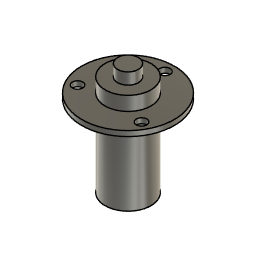
Slew_Bearing (Autodesk Fusion 360 archive; units mm, degrees)
design "GOCO bearing"
Autodesk Fusion 360 part; units mm, degrees
sketch "Sketch1" plane through (0, 0, 0) normal (0, 0, 1) x (1, 0, 0)
  circle A0 centre (0, 0) radius 22.25
  line L0 (0, 0) -> (0, 22.25) construction
  circle A1 centre (0, 17.75) radius 2.5
  line L1 (0, 17.75) -> (0, 20.25) construction
  circle A2 centre (-15.372, -8.875) radius 2.5
  circle A3 centre (15.372, -8.875) radius 2.5
  circle A4 centre (0, 0) radius 17.75 construction
  dimension "d1" = 44.5
  dimension "d2" = 5
  dimension "d3" = 2
  dimension "d5" = 360
  constraint coincident A0.centre L0.start
  constraint coincident A0 L0.end
  constraint vertical L0
  constraint coincident L0 A1.centre
  constraint coincident A1.centre L1.start
  constraint coincident L0 L1.end
  constraint coincident A1 L1.end
  constraint coincident A1.centre A4
  measures "d1" diameter of A0
  measures "d2" diameter of A1
  measures "d3" distance of L0.end L1.end
extrude "Extrude1" add sketch "Sketch1" along normal blind 2.5 makes body 1
sketch "Sketch2" plane through (0, 0, 2.5) normal (0, 0, 1) x (-1, 0, 0)
  circle A0 centre (0, -17.75) radius 2.5
  circle A1 centre (15.372, 8.875) radius 2.5
  circle A2 centre (-15.372, 8.875) radius 2.5
  circle A3 centre (0, 0) radius 22.25
  circle A4 centre (0, 0) radius 11
  dimension "d8" = 22
  constraint coincident A3.centre A4.centre
  measures "d8" diameter of A4
extrude "Extrude2" add sketch "Sketch2" along normal blind 6.7 contours A4 bodies 1
sketch "Sketch3" plane through (0, 0, 9.2) normal (0, 0, 1) x (-1, 0, 0)
  circle A0 centre (0, 0) radius 11
  circle A1 centre (0, 0) radius 5
  dimension "d11" = 10
  constraint coincident A0.centre A1.centre
  measures "d11" diameter of A1
extrude "Extrude3" add sketch "Sketch3" along normal blind 5.5 contours A1 bodies 1
sketch "Sketch4" plane through (0, 0, 0) normal (0, 0, -1) x (1, 0, 0)
  circle A0 centre (0, -17.75) radius 2.5
  circle A1 centre (-15.372, 8.875) radius 2.5
  circle A2 centre (15.372, 8.875) radius 2.5
  circle A3 centre (0, 0) radius 22.25
  circle A4 centre (0, 0) radius 11
  dimension "d14" = 22
  constraint coincident A3.centre A4.centre
  measures "d14" diameter of A4
extrude "Extrude4" add sketch "Sketch4" along normal blind 39 contours A4 bodies 1
copy_body "Body->Comp1" bodies 1 removing the originals makes body 2 in component "Component"
component "Component" placed x (1, 0, 0) y (0, 1, 0) z (0, 0, 1) at (0, 0, 0)
